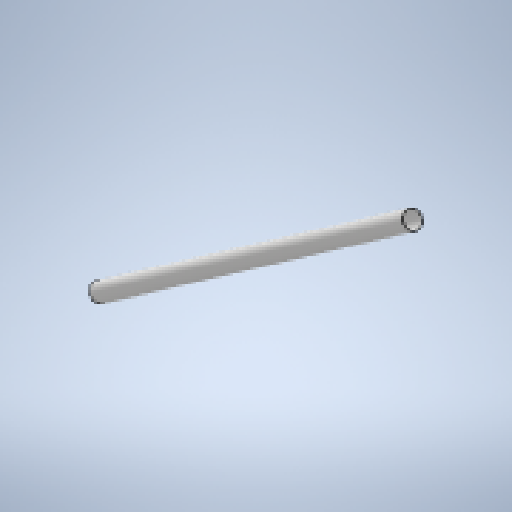
# Autodesk Inventor part: NDM-VOS dummy5
Saved by Autodesk Inventor 2025 (Build 290162010, 162A)
## iProperties
Created: 2024-10-01
Part Number: NDM-VOS dummy5
Material: Generic
Document SubType Name: Modeling
Designer: pokla
Density: 1 g/cm^3
Appearance: Default
Author: pokla
Autodesk Inventor part; units mm, degrees
ref_plane "YZ Plane" through (0, 0, 0) normal (1, 0, 0) x (0, 1, 0)
ref_plane "XZ Plane" through (0, 0, 0) normal (0, 1, 0) x (-1, 0, 0)
ref_plane "XY Plane" through (0, 0, 0) normal (0, 0, 1) x (1, 0, 0)
sketch "Sketch2" plane through (0, 0, 0) normal (0, 1, 0) x (-1, 0, 0)
  line L0 (0, 0) -> (0, 1300) construction
  line L1 (0, 1300) -> (-1802.1345, 2561.8682)
  line L2 (0, 1300) -> (-2200, 1300) construction
  dimension "d3" = 35
  dimension "d4" = 2200
  dimension "d5" = 1300
  constraints: 6 end point, 1 equal length, 1 horizontal, 1 vertical
  measures "d3" angle of L2 L1
  measures "d4" distance of L0.end L1.end
  measures "d5" distance of L0.start L0.end
ref_plane "Work Plane1" through (0, 0, 1300) normal (0.819152, 0, 0.5735764) x (0, 1, 0)
sketch "Sketch3" plane through (0, 0, 1300) normal (0.819152, 0, 0.5735764) x (0, 1, 0)
  circle A0 centre (0, 0) radius 50
  circle A1 centre (0, 0) radius 47
  point P0 (0, -1064.8977)
  point P1 (0, 0)
  dimension "d6" = 100
  dimension "d7" = 3
  constraints: 2 centre point, 1 coincident
  measures "d6" diameter of A0
  measures "d7" radial gap between concentric circles of A0 A1
sweep "Sweep1" add profiles "Sketch3" path "Sketch2"
body "Solid2"
